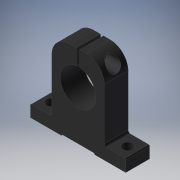
# Autodesk Inventor part: C-SHA30_b
Saved by Autodesk Inventor 2019 (Build 230136000, 136)
## iProperties
Created: 2022-11-16
Part Number: C-SHA30_b
Material: Generic
Catalog Web Link: www.cadenas.de
Description: C-SHA_base-Economy Shaft Supports - T-Shaped/Slit
Vendor: MISUMI
Document SubType Name: Modeling
Designer: psAdmin
Manufacturer: MISUMI
Mass: 48.6779 g
Surface Area: 141.331 cm^2
Volume: 48.6779 cm^3
Density: 1 g/cm^3
Appearance: PSOLRGB-175-175-175
Category: PARTsolutions
Company: MISUMI
Title: C-SHA30
Author: Cadenas PARTsolutions
Comments: Economy Shaft Supports - T-Shaped/Slit
PSOL_IDENT_0: {$CADENAS_DATA/23d-libs/misumi/metric/02_shaft_supports/c_sha/c_sha_base.prj},160 {VTYP=3D},{NB=C-SH
PSOL_IDENT_1: A30_b},{LINA=C-SHA30},{NN=C-SHA_base},{DATE=04.10.2022 06:54:53},{GEOMDATE=23.04.2021 02:46:37},{VER
PSOL_IDENT_2: SION=},{LINEID=60},{WBVAR=},{WBNUMERIC=}  {NB=C-SHA30_b},{LINA=C-SHA30},{KT=DUMMY},{PN=C-SHA30},{TYP
PSOL_IDENT_3: E=C-SHA},{D=30},{H=42},{H1=70},{T=20},{L1=64},{DD=9.0},{E=21.0},{S=10},{R=15},{L=80},{B=28},{W=44},{
PSOL_IDENT_4: M=M6},{R2=2},{W2=2.5},{M3D=6},{M3D2=13.5},{M3D3=11},{M3D4=6.4},{LB=20}
NB: C-SHA30_b
NN: C-SHA_base
NT: Economy Shaft Supports - T-Shaped/Slit
NBSYN: $PN._b
LINA: C-SHA30
CATALOG: Misumi
PN: C-SHA30
D: 30
H: 42
H1: 70
T: 20
L1: 64
DD: 9
E: 21
S: 10
R: 15
L: 80
B: 28
W: 44
M: M6
SUPPLIER: MISUMI
ARTICLENO: C-SHA30_b
BOMINFO: C-SHA30
CREATOR: CADENAS GmbH
Autodesk Inventor part; units mm, degrees
ref_plane "YZ Plane" through (0, 0, 0) normal (1, 0, 0) x (0, 1, 0)
ref_plane "XZ Plane" through (0, 0, 0) normal (0, 1, 0) x (-1, 0, 0)
ref_plane "XY Plane" through (0, 0, 0) normal (0, 0, 1) x (1, 0, 0)
sketch "_____1" plane through (0, 0, 0) normal (0, 0, 1) x (1, 0, 0)
  line L0 (-40, -33) -> (-40, -42)
  line L1 (-40, -42) -> (-14, -42)
  arc A0 (-13, -41) -> (-14, -42) centre (-13, -42) ccw
  line L2 (-13, -41) -> (13, -41)
  arc A1 (14, -42) -> (13, -41) centre (13, -42) ccw
  line L3 (14, -42) -> (40, -42)
  line L4 (40, -42) -> (40, -33)
  arc A2 (40, -33) -> (39, -32) centre (39, -33) ccw
  line L5 (39, -32) -> (24, -32)
  arc A3 (22, -30) -> (24, -32) centre (24, -30) ccw
  line L6 (22, -30) -> (22, 13)
  arc A4 (22, 13) -> (7, 28) centre (7, 13) ccw
  line L7 (7, 28) -> (-7, 28)
  arc A5 (-7, 28) -> (-22, 13) centre (-7, 13) ccw
  line L8 (-22, 13) -> (-22, -30)
  arc A6 (-24, -32) -> (-22, -30) centre (-24, -30) ccw
  line L9 (-24, -32) -> (-39, -32)
  arc A7 (-39, -32) -> (-40, -33) centre (-39, -33) ccw
  constraints: 20 end point, 16 point on circle, 8 centre point
extrude "Extrusion1" add sketch "_____1" along normal mid plane 20
sketch "_____2" plane through (0, 0, 0) normal (0, 0, 1) x (1, 0, 0)
  arc A0 (-1.25, 14.9478) -> (1.25, 14.9478) centre (0, 0) ccw
  line L0 (1.25, 14.9478) -> (1.25, 70)
  line L1 (1.25, 70) -> (-1.25, 70)
  line L2 (-1.25, 70) -> (-1.25, 14.9478)
  constraints: 6 end point, 2 point on circle, 1 centre point
extrude "Extrusion2" cut sketch "_____2" along normal mid plane 20
sketch "_____3" plane through (0, 0, 0) normal (0, 1, 0) x (1, 0, 0)
  circle A0 centre (32, 0) radius 4.5
  constraints: 1 centre point
extrude "Extrusion3" cut sketch "_____3" against normal blind 42
sketch "_____4" plane through (0, 0, 0) normal (0, 1, 0) x (1, 0, 0)
  circle A0 centre (-32, 0) radius 4.5
  constraints: 1 centre point
extrude "Extrusion4" cut sketch "_____4" against normal blind 42
sketch "_____5" plane through (0, 0, 0) normal (0, 0, 1) x (1, 0, 0)
  line L0 (50, 21) -> (-50, 21)
  line L1 (0, 21) -> (0, 24.2)
  line L2 (0, 24.2) -> (8.5, 24.2)
  line L3 (8.5, 24.2) -> (8.5, 26.5)
  line L4 (8.5, 26.5) -> (22, 26.5)
  line L5 (22, 26.5) -> (22, 21)
  line L6 (22, 21) -> (0, 21)
  constraints: 14 end point
revolve "Revolution1" cut sketch "_____5" angle 360 about axis through (50, 21, 0) along (1, 0, 0)
sketch "Sketch6" plane through (-1.25, 14.9478, 10) normal (1, 0, 0) x (0, 0, -1)
  point P0 (10, 6.0522)
hole "Hole1" at (-1.25, 21, 0) direction (-1, 0, 0) diameter 4.917 depth 20.75 countersink diameter 6 countersink angle 90 thread size "M6x1" class "6H" standard "ISO Metric profile"
ref_plane "to_bolt_XY" through (8.5, 21, 0) normal (1, 0, 0) x (0, 0, -1)
ref_plane "to_bolt_YZ" through (8.5, 21, 0) normal (0, 0, -1) x (0, 1, 0)
ref_plane "to_bolt_ZX" through (8.5, 21, 0) normal (0, 1, 0) x (1, 0, 0)
body "Solid1"
